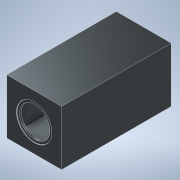
# Autodesk Inventor part: Фонарь
Saved by Autodesk Inventor 2021 (Build 250183000, 183)
## iProperties
Created: 2020-11-16
Part Number: Фонарь
Material: Чугун, серый
Document SubType Name: Modeling
Designer: Тимоха
Density: 7.15 g/cm^3
Appearance: Чугун серый
Mass: 419683 g
Surface Area: 55417.9 cm^2
Volume: 58696.9 cm^3
Author: Тимоха
Autodesk Inventor part; units mm, degrees
ref_plane "YZ Plane" through (0, 0, 0) normal (1, 0, 0) x (0, 1, 0)
ref_plane "XZ Plane" through (0, 0, 0) normal (0, 1, 0) x (-1, 0, 0)
ref_plane "XY Plane" through (0, 0, 0) normal (0, 0, 1) x (1, 0, 0)
sketch "Эскиз1" plane through (0, 0, 0) normal (0, 0, 1) x (1, 0, 0)
  line L0 (-270, 270) -> (-270, -270)
  line L1 (-270, -270) -> (270, -270)
  line L2 (270, -270) -> (270, 270)
  line L3 (270, 270) -> (-270, 270)
  line L4 (-270, 270) -> (270, -270) construction
  line L5 (-270, -270) -> (270, 270) construction
  line L6 (-230, -230) -> (-230, 230)
  line L7 (-230, 230) -> (230, 230)
  line L8 (230, 230) -> (230, -230)
  line L9 (230, -230) -> (-230, -230)
  line L10 (-230, -230) -> (230, 230) construction
  line L11 (-230, 230) -> (230, -230) construction
  point P0 (0, 0)
  dimension "d0" = 540
  dimension "d1" = 540
  dimension "d2" = 460
  dimension "d3" = 460
  constraints: 24 end point, 5 parallel, 4 midpoint, 2 perpendicular, 1 vertical
  measures "d0" distance of L0.start L0.end
  measures "d1" distance of L1.end L0.end
  measures "d2" distance of L6.start L6.end
  measures "d3" distance of L6.end L7.end
extrude "Выдавливание1" add sketch "Эскиз1" along normal blind 20 contours L3 L2 L1 L0 | L6 L7 L8 L9
sketch "Эскиз2" plane through (0, 0, 20) normal (0, 0, 1) x (1, 0, 0)
  line L0 (-250, -250) -> (-250, 250)
  line L1 (-250, 250) -> (250, 250)
  line L2 (250, 250) -> (250, -250)
  line L3 (250, -250) -> (-250, -250)
  line L4 (-250, -250) -> (250, 250) construction
  line L5 (-250, 250) -> (250, -250) construction
  line L6 (270, 270) -> (-270, 270) projected
  line L7 (-270, 270) -> (-270, -270) projected
  line L8 (-270, -270) -> (270, -270) projected
  line L9 (270, -270) -> (270, 270) projected
  point P0 (0, 0)
  dimension "d6" = 500
  dimension "d7" = 500
  constraints: 12 end point, 2 midpoint, 2 parallel, 1 perpendicular, 1 vertical
  measures "d6" distance of L0.start L0.end
  measures "d7" distance of L0.end L1.end
extrude "Выдавливание2" add sketch "Эскиз2" along normal blind 500
sketch "Эскиз3" plane through (0, 0, 0) normal (0, 0, -1) x (-1, 0, 0)
  circle A0 centre (0, 0) radius 240
  circle A1 centre (0, 0) radius 200
  dimension "d10" = 480
  dimension "d11" = 400
  constraints: 2 centre point, 2 coincident
  measures "d10" diameter of A0
  measures "d11" diameter of A1
extrude "Выдавливание3" add sketch "Эскиз3" along normal blind 20
sketch "Эскиз4" plane through (0, 0, 0) normal (0, 0, -1) x (-1, 0, 0)
  circle A0 centre (0, 0) radius 200 projected
extrude "Выдавливание4" cut sketch "Эскиз4" against normal blind 200
sketch "Эскиз5" plane through (0, 0, -20) normal (0, 0, -1) x (-1, 0, 0)
  circle A0 centre (0, 0) radius 200 projected
  circle A1 centre (0, 0) radius 200 projected
  line L0 (0, 200) -> (0, 220)
  dimension "d16" = 20
  constraints: 2 end point, 1 vertical, 1 vertical alignment, 1 other
  measures "d16" distance of L0.start L0.end
hole "Отверстие1" at (0, 220, -20) direction (0, 0, 1) diameter 22 end through all
pattern_circular "Круговой массив1" count 12 over 360 about axis through (0, 0, 0) along (0, 0, -1) of "Отверстие1"
sketch "Эскиз6" plane through (0, 0, 520) normal (0, 0, 1) x (1, 0, 0)
  line L0 (-270, 270) -> (-270, -270) projected
  line L1 (270, 270) -> (-270, 270) projected
  line L2 (-270, -270) -> (270, -270) projected
  line L3 (270, -270) -> (270, 270) projected
  point P0 (0, 0)
extrude "Выдавливание5" add sketch "Эскиз6" along normal blind 30
sketch "Эскиз7" plane through (0, 0, 550) normal (0, 0, 1) x (1, 0, 0)
  circle A0 centre (0, 0) radius 150
  dimension "d29" = 300
  constraints: 1 centre point, 1 coincident
  measures "d29" diameter of A0
extrude "Выдавливание6" cut sketch "Эскиз7" against normal blind 31
sketch "Эскиз8" plane through (0, 0, 550) normal (0, 0, 1) x (1, 0, 0)
  line L0 (-250, -250) -> (-250, 250)
  line L1 (-250, 250) -> (250, 250)
  line L2 (250, 250) -> (250, -250)
  line L3 (250, -250) -> (-250, -250)
  line L4 (-250, -250) -> (250, 250) construction
  line L5 (-250, 250) -> (250, -250) construction
  line L6 (-270, 270) -> (-270, -270) projected
  line L7 (270, 270) -> (-270, 270) projected
  line L8 (-270, -270) -> (270, -270) projected
  line L9 (270, -270) -> (270, 270) projected
  point P0 (0, 0)
  dimension "d32" = 500
  dimension "d33" = 500
  constraints: 12 end point, 2 midpoint, 2 parallel, 1 perpendicular, 1 vertical
  measures "d32" distance of L0.start L0.end
  measures "d33" distance of L0.end L1.end
extrude "Выдавливание7" add sketch "Эскиз8" along normal blind 500
sketch "Эскиз9" plane through (0, 0, 1050) normal (0, 0, 1) x (1, 0, 0)
  line L0 (-270, 270) -> (-270, -270) projected
  line L1 (270, 270) -> (-270, 270) projected
  line L2 (270, -270) -> (270, 270) projected
  line L3 (-270, -270) -> (270, -270) projected
  point P0 (0, 0)
extrude "Выдавливание8" add sketch "Эскиз9" along normal blind 30
sketch "Эскиз10" plane through (0, 0, 1080) normal (0, 0, 1) x (1, 0, 0)
  circle A0 centre (0, 0) radius 150
  dimension "d38" = 300
  constraints: 1 centre point, 1 coincident
  measures "d38" diameter of A0
extrude "Выдавливание9" cut sketch "Эскиз10" against normal blind 30
sketch "Эскиз11" plane through (0, 0, 550) normal (0, 0, 1) x (1, 0, 0)
  circle A0 centre (0, 0) radius 175
  circle A1 centre (0, 0) radius 150 projected
  dimension "d41" = 350
  constraints: 1 centre point, 1 coincident
  measures "d41" diameter of A0
extrude "Выдавливание10" cut sketch "Эскиз11" against normal blind 5
fillet "Сопряжение1" radius 2 1 edges at (-175, 0, 545)
sketch "Эскиз12" plane through (0, 0, 520) normal (0, 0, -1) x (-1, 0, 0)
  circle A0 centre (0, 0) radius 150 projected
  circle A1 centre (0, 0) radius 165
  dimension "d45" = 330
  constraints: 1 centre point, 1 coincident
  measures "d45" diameter of A1
extrude "Выдавливание11" cut sketch "Эскиз12" against normal blind 5
fillet "Сопряжение2" radius 2 1 edges at (165, 0, 525)
sketch "Эскиз13" plane through (0, 0, 1080) normal (0, 0, 1) x (1, 0, 0)
  circle A0 centre (0, 0) radius 150 projected
  circle A1 centre (0, 0) radius 175
  dimension "d49" = 350
  constraints: 1 centre point, 1 coincident
  measures "d49" diameter of A1
extrude "Выдавливание12" cut sketch "Эскиз13" against normal blind 5
sketch "Эскиз14" plane through (0, 0, 1050) normal (0, 0, -1) x (-1, 0, 0)
  circle A0 centre (0, 0) radius 150 projected
  circle A1 centre (0, 0) radius 165
  dimension "d52" = 330
  constraints: 1 centre point, 1 coincident
  measures "d52" diameter of A1
extrude "Выдавливание13" cut sketch "Эскиз14" against normal blind 5
fillet "Сопряжение3" radius 2 2 edges at (165, 0, 1055) (-175, 0, 1075)
